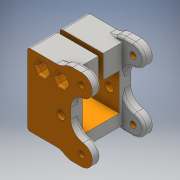
# Autodesk Inventor part: arm_socket
Saved by Autodesk Inventor 2016 (Build 200138000, 138)
## iProperties
Created: 2016-10-27
Part Number: arm_socket
Material: Generic
Document SubType Name: Modeling
Designer: Jakub
Density: 1 g/cm^3
Appearance: Default
Mass: 8.53964 g
Surface Area: 52.0512 cm^2
Volume: 8.53964 cm^3
Author: Jakub
Autodesk Inventor part; units mm, degrees
ref_plane "YZ Plane" through (0, 0, 0) normal (1, 0, 0) x (0, 1, 0)
ref_plane "XZ Plane" through (0, 0, 0) normal (0, 1, 0) x (-1, 0, 0)
ref_plane "XY Plane" through (0, 0, 0) normal (0, 0, 1) x (1, 0, 0)
sketch "Sketch1" plane through (0, 0, 0) normal (1, 0, 0) x (0, 1, 0)
  line L0 (-12.5, 15) -> (12.5, 15)
  line L1 (12.5, 15) -> (12.5, -15)
  line L2 (12.5, -15) -> (-12.5, -15)
  line L3 (-12.5, -15) -> (-12.5, 15)
  line L4 (-12.5, 15) -> (12.5, -15) construction
  line L5 (12.5, 15) -> (-12.5, -15) construction
  line L6 (-7.65, 5.3) -> (7.65, 5.3)
  line L7 (7.65, 5.3) -> (7.65, -10)
  line L8 (7.65, -10) -> (-7.65, -10)
  line L9 (-7.65, -10) -> (-7.65, 5.3)
  line L10 (-7.65, 5.3) -> (7.65, -10) construction
  line L11 (7.65, 5.3) -> (-7.65, -10) construction
  line L12 (0, 5.3) -> (1, 5.3)
  line L13 (1, 5.3) -> (-1, 5.3)
  line L14 (-1, 5.3) -> (-1, 15)
  line L15 (-1, 15) -> (1, 15)
  line L16 (1, 15) -> (1, 5.3)
  point P0 (0, 0)
  point P1 (0, -2.35)
  dimension "d0" = 25
  dimension "d1" = 30
  dimension "d2" = 15.3
  dimension "d3" = 15.3
  dimension "d4" = 5
  dimension "d5" = 4.85
  dimension "d6" = 1
  dimension "d7" = 2
  constraints: 34 end point, 6 parallel, 5 midpoint, 3 horizontal, 3 perpendicular, 2 point on line
  measures "d0" distance of L1.end L2.end
  measures "d1" distance of L0.end L1.end
  measures "d2" distance of L7.end L8.end
  measures "d3" distance of L6.end L7.end
  measures "d4" distance between parallel lines of L2 L8
  measures "d5" distance between parallel lines of L1 L7
  measures "d6" distance of L12.start L12.end
  measures "d7" distance of L14.end L15.end
extrude "Extrusion1" add sketch "Sketch1" along normal blind 8 contours L0 L14 L6 L9 L8 L7 L16 L1 L2 L3
sketch "Sketch2" plane through (0, 12.5, 15) normal (0, 1, 0) x (1, 0, 0)
  line L0 (0, 0) -> (8, 0) projected
  line L1 (4, 0) -> (4, 5)
  circle A0 centre (4, 5) radius 1.25
  point P0 (0, 15)
  dimension "d10" = 5
  dimension "d11" = 2.5
  constraints: 2 end point, 1 centre point, 1 coincident, 1 midpoint, 1 vertical
  measures "d10" distance of L1.start L1.end
  measures "d11" diameter of A0
extrude "Extrusion2" cut sketch "Sketch2" against normal through all
sketch "Sketch3" plane through (0, 12.5, 15) normal (0, 1, 0) x (1, 0, 0)
  line L0 (0, 30) -> (8, 30) projected
  line L1 (4, 30) -> (4, 17.45)
  circle A0 centre (4, 17.45) radius 1.75
  point P0 (0, 15)
  dimension "d14" = 12.55
  dimension "d15" = 3.5
  constraints: 2 end point, 1 centre point, 1 coincident, 1 midpoint, 1 vertical
  measures "d14" distance of L1.start L1.end
  measures "d15" diameter of A0
extrude "Extrusion3" cut sketch "Sketch3" against normal through all
sketch "Sketch4" plane through (0, 12.5, 15) normal (0, 1, 0) x (1, 0, 0)
  circle A0 centre (4, 5) radius 1.25 projected
  circle A1 centre (4, 5) radius 2.5
  point P0 (0, 15)
  dimension "d18" = 5
  constraints: 1 centre point, 1 coincident
  measures "d18" diameter of A1
extrude "Extrusion4" cut sketch "Sketch4" against normal blind 5
sketch "Sketch5" plane through (0, -12.5, -15) normal (0, -1, 0) x (1, 0, 0)
  circle A0 centre (4, 25) radius 1.25 projected
  line L0 (2.8, 27.0785) -> (5.2, 27.0785)
  line L1 (5.2, 27.0785) -> (6.4, 25)
  line L2 (6.4, 25) -> (5.2, 22.9215)
  line L3 (5.2, 22.9215) -> (2.8, 22.9215)
  line L4 (2.8, 22.9215) -> (1.6, 25)
  line L5 (1.6, 25) -> (2.8, 27.0785)
  line L6 (0, 30) -> (8, 30) projected
  point P0 (0, 15)
  dimension "d21" = 2.4
  constraints: 12 end point, 1 coincident, 1 parallel, 13 other
  measures "d21" distance of L3.end L4.end
extrude "Extrusion5" cut sketch "Sketch5" against normal blind 5
fillet "Fillet1" radius 1 1 edges at (1.5, 12.5, 10)
fillet "Fillet2" radius 1 6 edges at (2.2, -12.5, 11.0392) (4, -12.5, 12.0785) (5.8, -12.5, 11.0392) (5.8, -12.5, 8.9608) (4, -12.5, 7.9215) (2.2, -12.5, 8.9608)
sketch "Sketch6" plane through (8, 0, 0) normal (1, 0, 0) x (0, 0, -1)
  line L0 (15, 12.5) -> (-15, 12.5) projected
  line L1 (-15, 12.5) -> (-10, 12.5)
  line L2 (-10, 12.5) -> (-10, 9)
  line L3 (-10, 9) -> (-15, 9)
  line L4 (-15, 9) -> (-15, 12.5)
  line L5 (15, 12.5) -> (10, 12.5)
  line L6 (10, 12.5) -> (10, 9)
  line L7 (10, 9) -> (15, 9)
  line L8 (15, 9) -> (15, 12.5)
  line L9 (-15, -12.5) -> (15, -12.5) projected
  line L10 (-15, -12.5) -> (-10, -12.5)
  line L11 (-10, -12.5) -> (-10, -9)
  line L12 (-10, -9) -> (-15, -9)
  line L13 (-15, -9) -> (-15, -12.5)
  line L14 (15, -12.5) -> (10, -12.5)
  line L15 (10, -12.5) -> (10, -9)
  line L16 (10, -9) -> (15, -9)
  line L17 (15, -9) -> (15, -12.5)
  point P0 (0, 0)
  dimension "d26" = 5
  dimension "d27" = 3.5
  dimension "d28" = 5
  dimension "d29" = 3.5
  dimension "d30" = 5
  dimension "d31" = 3.5
  dimension "d32" = 5
  dimension "d33" = 3.5
  constraints: 32 end point, 8 parallel, 4 horizontal, 4 perpendicular
  measures "d26" distance of L2.end L3.end
  measures "d27" distance of L1.end L2.end
  measures "d28" distance of L7.end L6.end
  measures "d29" distance of L6.end L5.end
  measures "d30" distance of L12.end L11.end
  measures "d31" distance of L11.end L10.end
  measures "d32" distance of L15.end L16.end
  measures "d33" distance of L14.end L15.end
extrude "Extrusion6" add sketch "Sketch6" along normal blind 7
fillet "Fillet3" radius 2.5 8 edges at (15, 10.75, 15) (15, 10.75, 10) (15, -10.75, 15) (15, -10.75, 10) (15, -10.75, -10) (15, -10.75, -15) (15, 10.75, -10) (15, 10.75, -15)
sketch "Sketch7" plane through (0, -12.5, -15) normal (0, -1, 0) x (1, 0, 0)
  arc A0 (12.5, 25) -> (12.5, 30) centre (12.5, 27.5) ccw projected
  circle A1 centre (12.5, 27.5) radius 1.25
  arc A2 (12.5, 0) -> (12.5, 5) centre (12.5, 2.5) ccw projected
  circle A3 centre (12.5, 2.5) radius 1.25
  point P0 (0, 15)
  dimension "d37" = 2.5
  dimension "d38" = 2.5
  constraints: 2 centre point, 2 coincident
  measures "d37" diameter of A1
  measures "d38" diameter of A3
extrude "Extrusion7" cut sketch "Sketch7" against normal through all
sketch "Sketch8" plane through (0, 0, 0) normal (-1, 0, 0) x (0, 0, 1)
  line L0 (5.3, 1) -> (5.3, 7.65) projected
  line L1 (5.3, 1) -> (5.3, 7.65)
  line L2 (-10, 7.65) -> (5.3, 7.65) projected
  line L3 (5.3, 7.65) -> (-10, 7.65)
  line L4 (-10, -7.65) -> (-10, 7.65) projected
  line L5 (-10, 7.65) -> (-10, -7.65)
  line L6 (5.3, -7.65) -> (-10, -7.65) projected
  line L7 (-10, -7.65) -> (5.3, -7.65)
  line L8 (5.3, -1) -> (5.3, -7.65) projected
  line L9 (5.3, -7.65) -> (5.3, -1)
  line L10 (15, -1) -> (15, -12.5) projected
  line L11 (5.3, -1) -> (15, -1)
  line L12 (15, -1) -> (15, -12.5)
  line L13 (15, -12.5) -> (-15, -12.5) projected
  line L14 (15, -12.5) -> (-15, -12.5)
  line L15 (-15, -12.5) -> (-15, 12.5) projected
  line L16 (-15, -12.5) -> (-15, 12.5)
  line L17 (10, 12.5) -> (15, 12.5) projected
  line L18 (-15, 12.5) -> (15, 12.5)
  line L19 (15, -1) -> (15, 1) projected
  line L20 (15, 12.5) -> (15, 1)
  line L21 (15, 1) -> (5.3, 1)
  point P0 (0, 0)
  point P1 (15, 7)
  constraints: 24 end point, 7 collinear, 5 perpendicular
extrude "Extrusion8" add sketch "Sketch8" along normal blind 10 contours L0 L2 L4 L6 L8 L11 L10 L13 L15 L18 L17 L20 L21
pattern_linear "Rectangular Pattern1" count 2 spacing 8 along (-1, 0, 0) of "Extrusion2", "Extrusion5", "Fillet2", "Extrusion4", "Fillet1"
sketch "Sketch10" plane through (8, -12.5, 10) normal (0, 0, -1) x (-1, 0, 0)
  line L0 (0, 3.5) -> (-4.5, 3.5) projected
  line L1 (-4.5, 0) -> (-4.5, 3.5) projected
  line L2 (0, 3.5) -> (-4.5, 3.5)
  line L3 (-4.5, 3.5) -> (-4.5, 0)
  line L4 (-4.5, 0) -> (0, 0)
  line L5 (0, 0) -> (0, 3.5)
  line L6 (-4.5, 21.5) -> (-4.5, 25) projected
  line L7 (0, 21.5) -> (-4.5, 21.5)
  line L8 (-4.5, 21.5) -> (-4.5, 25)
  line L9 (-4.5, 25) -> (0, 25)
  line L10 (0, 25) -> (0, 21.5)
  point P0 (8, 12.5)
  constraints: 16 end point, 4 parallel, 2 horizontal, 2 perpendicular
extrude "Extrusion9" add sketch "Sketch10" along normal blind 2
sketch "Sketch11" plane through (8, -12.5, -10) normal (0, 0, 1) x (1, 0, 0)
  line L0 (4.5, 3.5) -> (4.5, 0) projected
  line L1 (4.5, 0) -> (0, 0)
  line L2 (0, 0) -> (0, 3.5)
  line L3 (0, 3.5) -> (4.5, 3.5)
  line L4 (4.5, 3.5) -> (4.5, 0)
  line L5 (4.5, 25) -> (4.5, 21.5) projected
  line L6 (0, 25) -> (4.5, 25) projected
  line L7 (4.5, 21.5) -> (0, 21.5)
  line L8 (0, 21.5) -> (0, 25)
  line L9 (0, 25) -> (4.5, 25)
  line L10 (4.5, 25) -> (4.5, 21.5)
  point P0 (-8, 12.5)
  constraints: 16 end point, 4 parallel, 2 horizontal, 2 perpendicular
extrude "Extrusion10" add sketch "Sketch11" along normal blind 2
sketch "Sketch12" plane through (8, -9, 15) normal (0, 0, 1) x (1, 0, 0)
  line L0 (4.5, -3.5) -> (4.5, 0) projected
  line L1 (4.5, 0) -> (-1.5, 0)
  line L2 (-1.5, 0) -> (-1.5, -3.5)
  line L3 (-1.5, -3.5) -> (4.5, -3.5)
  line L4 (4.5, -3.5) -> (4.5, 0)
  line L5 (4.5, 18) -> (4.5, 21.5) projected
  line L6 (4.5, 21.5) -> (-1.5, 21.5)
  line L7 (-1.5, 21.5) -> (-1.5, 18)
  line L8 (-1.5, 18) -> (4.5, 18)
  line L9 (4.5, 18) -> (4.5, 21.5)
  point P0 (-8, 9)
  dimension "d60" = 6
  dimension "d61" = 6
  constraints: 16 end point, 4 parallel, 2 horizontal, 2 perpendicular
  measures "d60" distance of L3.end L2.end
  measures "d61" distance of L8.end L7.end
extrude "Extrusion11" add sketch "Sketch12" along normal blind 2
sketch "Sketch13" plane through (8, -9, -15) normal (0, 0, -1) x (-1, 0, 0)
  line L0 (-4.5, -3.5) -> (-4.5, 0) projected
  line L1 (-4.5, -3.5) -> (1.5, -3.5)
  line L2 (1.5, -3.5) -> (1.5, 0)
  line L3 (1.5, 0) -> (-4.5, 0)
  line L4 (-4.5, 0) -> (-4.5, -3.5)
  line L5 (-4.5, 18) -> (-4.5, 21.5) projected
  line L6 (-4.5, 21.5) -> (1.5, 21.5)
  line L7 (1.5, 21.5) -> (1.5, 18)
  line L8 (1.5, 18) -> (-4.5, 18)
  line L9 (-4.5, 18) -> (-4.5, 21.5)
  point P0 (8, 9)
  dimension "d64" = 6
  dimension "d65" = 6
  constraints: 16 end point, 4 parallel, 2 horizontal, 2 perpendicular
  measures "d64" distance of L3.end L2.end
  measures "d65" distance of L7.end L8.end
extrude "Extrusion12" add sketch "Sketch13" along normal blind 2
sketch "Sketch14" plane through (-10, -12.5, -11) normal (0, -1, 0) x (1, 0, 0)
  line L0 (22.5, -6) -> (16.5, -6) projected
  line L1 (22.5, 1) -> (22.5, 3) projected
  arc A0 (22.5, -6) -> (22.5, 3) centre (22.5, -1.5) ccw
  line L2 (18, 19) -> (22.5, 19) projected
  line L3 (22.5, 26) -> (22.5, 28) projected
  arc A1 (22.5, 19) -> (22.5, 28) centre (22.5, 23.5) ccw
  line L4 (22.5, -4) -> (22.5, -6) projected
  line L5 (22.5, -6) -> (22.5, -4)
  line L6 (22.5, 1) -> (22.5, 3)
  arc A2 (22.5, -4) -> (22.5, 1) centre (22.5, -1.5) ccw
  line L7 (22.5, 21) -> (22.5, 19) projected
  line L8 (22.5, 19) -> (22.5, 21)
  line L9 (16.5, 28) -> (22.5, 28) projected
  line L10 (22.5, 28) -> (22.5, 26)
  arc A3 (22.5, 21) -> (22.5, 26) centre (22.5, 23.5) ccw
  point P0 (10, 11)
  dimension "d68" = 4.5
  dimension "d69" = 4.5
  constraints: 8 end point, 8 point on circle, 4 centre point, 3 collinear, 1 vertical
  measures "d68" radius of A0
  measures "d69" radius of A1
extrude "Extrusion13" add sketch "Sketch14" against normal blind 3.5
sketch "Sketch15" plane through (-10, 12.5, 11) normal (0, 1, 0) x (1, 0, 0)
  line L0 (22.5, 21) -> (22.5, 19) projected
  line L1 (22.5, 28) -> (16.5, 28) projected
  arc A0 (22.5, 19) -> (22.5, 28) centre (22.5, 23.5) ccw
  arc A1 (22.5, 21) -> (22.5, 26) centre (22.5, 23.5) ccw projected
  arc A2 (22.5, 21) -> (22.5, 26) centre (22.5, 23.5) ccw
  arc A3 (22.5, -6) -> (22.5, 3) centre (22.5, -1.5) ccw projected
  arc A4 (22.5, -6) -> (22.5, 3) centre (22.5, -1.5) ccw
  arc A5 (22.5, -4) -> (22.5, 1) centre (22.5, -1.5) ccw projected
  line L2 (22.5, 1) -> (22.5, 3) projected
  arc A6 (22.5, -4) -> (22.5, 1) centre (22.5, -1.5) ccw
  line L3 (22.5, 26) -> (22.5, 28) projected
  line L4 (22.5, 28) -> (22.5, 26)
  line L5 (22.5, 21) -> (22.5, 19)
  line L6 (22.5, 3) -> (22.5, 1)
  line L7 (22.5, -4) -> (22.5, -6) projected
  line L8 (22.5, -4) -> (22.5, -6)
  point P0 (10, 11)
  constraints: 8 end point, 8 point on circle, 4 centre point, 2 collinear, 2 vertical
extrude "Extrusion14" add sketch "Sketch15" against normal blind 3.5
fillet "Fillet11" radius 6 8 edges at (6.5, -10.75, -17) (6.5, -10.75, -15) (6.5, 10.75, -17) (6.5, 10.75, -15) (6.5, 10.75, 15) (6.5, 10.75, 17) (6.5, -10.75, 15) (6.5, -10.75, 17)
fillet "Fillet12" radius 6 4 edges at (8, -10.75, -8) (8, 10.75, -8) (8, -10.75, 8) (8, 10.75, 8)
fillet "Fillet13" radius 1 20 edges at (6.9291, -9, 16.7446) (3.7599, -9, 15.2554) (16.9884, -9, 12.8223) (9.4644, -9, 6.0356) (10.5806, -9, 17) (10.5806, -9, -17) (6.9291, -9, -16.7446) (3.7599, -9, -15.2554) (9.4644, -9, -6.0356) (16.9884, -9, -12.8223) (16.9884, 9, -12.8223) (10.5806, 9, -17) (6.9291, 9, -16.7446) (3.7599, 9, -15.2554) (9.4644, 9, -6.0356) (16.9884, 9, 12.8223) (10.5806, 9, 17) (6.9291, 9, 16.7446) (3.7599, 9, 15.2554) (9.4644, 9, 6.0356)
fillet "Fillet14" radius 1 3 edges at (-10, 0, -15) (-10, -6.75, 15) (-10, 6.75, 15)
equation "\"d19\" = d18"
body "Solid1"
